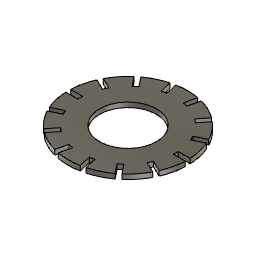
Assembly_file (Autodesk Fusion 360 archive; units mm, degrees)
design "Hringur_Litill"
Autodesk Fusion 360 part; units mm, degrees
sketch "Sketch1" plane through (0, 0, 0) normal (0, 0, 1) x (1, 0, 0)
  circle A0 centre (0, 0) radius 23.75
  line L0 (49.96, 2) -> (39.96, 2)
  line L1 (39.96, 2) -> (39.96, -2)
  line L2 (39.96, -2) -> (49.96, -2)
  line L3 (44.1446, 23.4788) -> (35.1349, 19.1399)
  line L4 (36.8705, 15.536) -> (45.8802, 19.8749)
  line L5 (35.1349, 19.1399) -> (36.8705, 15.536)
  line L6 (29.5859, 40.3073) -> (23.351, 32.489)
  line L7 (26.4783, 29.995) -> (32.7132, 37.8133)
  line L8 (23.351, 32.489) -> (26.4783, 29.995)
  line L9 (9.1673, 49.1524) -> (6.9421, 39.4031)
  line L10 (10.8418, 38.5131) -> (13.067, 48.2623)
  line L11 (6.9421, 39.4031) -> (10.8418, 38.5131)
  line L12 (-13.067, 48.2623) -> (-10.8418, 38.5131)
  line L13 (-6.9421, 39.4031) -> (-9.1673, 49.1524)
  line L14 (-10.8418, 38.5131) -> (-6.9421, 39.4031)
  line L15 (-32.7132, 37.8133) -> (-26.4783, 29.995)
  line L16 (-23.351, 32.489) -> (-29.5859, 40.3073)
  line L17 (-26.4783, 29.995) -> (-23.351, 32.489)
  line L18 (-45.8802, 19.8749) -> (-36.8705, 15.536)
  line L19 (-35.1349, 19.1399) -> (-44.1446, 23.4788)
  line L20 (-36.8705, 15.536) -> (-35.1349, 19.1399)
  line L21 (-49.96, -2) -> (-39.96, -2)
  line L22 (-39.96, 2) -> (-49.96, 2)
  line L23 (-39.96, -2) -> (-39.96, 2)
  line L24 (-44.1446, -23.4788) -> (-35.1349, -19.1399)
  line L25 (-36.8705, -15.536) -> (-45.8802, -19.8749)
  line L26 (-35.1349, -19.1399) -> (-36.8705, -15.536)
  line L27 (-29.5859, -40.3073) -> (-23.351, -32.489)
  line L28 (-26.4783, -29.995) -> (-32.7132, -37.8133)
  line L29 (-23.351, -32.489) -> (-26.4783, -29.995)
  line L30 (-9.1673, -49.1524) -> (-6.9421, -39.4031)
  line L31 (-10.8418, -38.5131) -> (-13.067, -48.2623)
  line L32 (-6.9421, -39.4031) -> (-10.8418, -38.5131)
  line L33 (13.067, -48.2623) -> (10.8418, -38.5131)
  line L34 (6.9421, -39.4031) -> (9.1673, -49.1524)
  line L35 (10.8418, -38.5131) -> (6.9421, -39.4031)
  line L36 (32.7132, -37.8133) -> (26.4783, -29.995)
  line L37 (23.351, -32.489) -> (29.5859, -40.3073)
  line L38 (26.4783, -29.995) -> (23.351, -32.489)
  line L39 (45.8802, -19.8749) -> (36.8705, -15.536)
  line L40 (35.1349, -19.1399) -> (44.1446, -23.4788)
  line L41 (36.8705, -15.536) -> (35.1349, -19.1399)
  arc A1 (49.96, 2) -> (45.8802, 19.8749) centre (0, 0) ccw
  arc A2 (44.1446, 23.4788) -> (32.7132, 37.8133) centre (0, 0) ccw
  arc A3 (29.5859, 40.3073) -> (13.067, 48.2623) centre (0, 0) ccw
  arc A4 (9.1673, 49.1524) -> (-9.1673, 49.1524) centre (0, 0) ccw
  arc A5 (-13.067, 48.2623) -> (-29.5859, 40.3073) centre (0, 0) ccw
  arc A6 (-32.7132, 37.8133) -> (-44.1446, 23.4788) centre (0, 0) ccw
  arc A7 (-45.8802, 19.8749) -> (-49.96, 2) centre (0, 0) ccw
  arc A8 (-49.96, -2) -> (-45.8802, -19.8749) centre (0, 0) ccw
  arc A9 (-44.1446, -23.4788) -> (-32.7132, -37.8133) centre (0, 0) ccw
  arc A10 (-29.5859, -40.3073) -> (-13.067, -48.2623) centre (0, 0) ccw
  arc A11 (-9.1673, -49.1524) -> (9.1673, -49.1524) centre (0, 0) ccw
  arc A12 (13.067, -48.2623) -> (29.5859, -40.3073) centre (0, 0) ccw
  arc A13 (32.7132, -37.8133) -> (44.1446, -23.4788) centre (0, 0) ccw
  arc A14 (45.8802, -19.8749) -> (49.96, -2) centre (0, 0) ccw
  dimension "d1" = 100
  dimension "d6" = 47.5
  dimension "d7" = 10
  dimension "d8" = 10
  dimension "d9" = 4
  dimension "d11" = 360
  constraint coincident A0.centre A1.centre
  constraint horizontal L0
  constraint perpendicular L0 L1
  constraint perpendicular L1 L2
  constraint concentric A1 A2
  constraint concentric A2 A3
  constraint concentric A3 A4
  constraint concentric A4 A5
  constraint concentric A5 A6
  constraint concentric A6 A7
  constraint concentric A7 A8
  constraint concentric A8 A9
  constraint concentric A9 A10
  constraint concentric A10 A11
  constraint concentric A11 A12
  constraint concentric A12 A13
  constraint concentric A13 A14
  measures "d1" diameter of A1
  measures "d6" diameter of A0
  measures "d7" distance of L0.start L0.end
  measures "d8" distance of L1.end L2.end
  measures "d9" distance of L0.end L1.end
extrude "Extrude1" add sketch "Sketch1" along normal blind 4
equation "d1 = D_o"
equation "D_o = 100 mm"
equation "D_i = 47.5 mm"
equation "þykkt = 4 mm"
equation "offset = 10 mm"
equation "d6 = D_i"
equation "d7 = offset"
equation "d8 = offset"
equation "d9 = þykkt"
equation "d12 = þykkt"

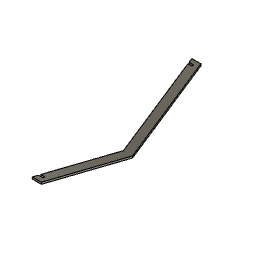
design "Lampi1"
Autodesk Fusion 360 part; units mm, degrees
sketch "Sketch1" plane through (0, 0, 0) normal (0, 0, 1) x (1, 0, 0)
  line L0 (0, 0) -> (20, 0)
  line L1 (20, 0) -> (120, -250)
  line L2 (120, -250) -> (70, -400)
  line L3 (70, -400) -> (50, -400)
  line L4 (4, -10) -> (14, -10)
  line L5 (53.3333, -390) -> (63.3333, -390)
  line L6 (63.3333, -386) -> (54.6667, -386)
  line L7 (100, -250) -> (54.6667, -386)
  line L8 (53.3333, -390) -> (50, -400)
  line L9 (0, 0) -> (4, -10)
  line L10 (5.6, -14) -> (100, -250)
  line L11 (14, -10) -> (14, -14)
  line L12 (5.6, -14) -> (14, -14)
  line L13 (63.3333, -390) -> (63.3333, -386)
  dimension "d4" = 400
  dimension "d5" = 50
  dimension "d6" = 50
  dimension "d7" = 250
  dimension "d9" = 20
  dimension "d10" = 20
  dimension "d11" = 20
  dimension "d12" = 10
  dimension "d13" = 4
  dimension "d14" = 10
  dimension "d15" = 10
  dimension "d16" = 4
  dimension "d17" = 10
  dimension "d27" = 4
  constraint coincident L0.start L9.start
  constraint horizontal L0
  constraint parallel L0 L3
  constraint parallel L1 L9
  constraint parallel L0 L4
  constraint coincident L10.start L9
  constraint coincident L5.start L7
  constraint parallel L3 L5
  constraint parallel L5 L6
  constraint collinear L7 L8
  constraint collinear L9 L10
  constraint perpendicular L11 L12
  constraint perpendicular L6 L13
  measures "d4" vertical distance of L0.start L3.end
  measures "d5" horizontal distance of L7.start L3.end
  measures "d6" horizontal distance of L0.start L3.end
  measures "d7" vertical distance of L0.start L7.start
  measures "d9" distance of L0.start L0.end
  measures "d10" distance of L7.start L1.end
  measures "d11" horizontal distance of L3.end L2.end
  measures "d12" vertical distance of L0.start L4.start
  measures "d13" vertical distance of L4.start L10.start
  measures "d14" distance of L4.start L4.end
  measures "d15" vertical distance of L3.end L5.start
  measures "d16" vertical distance of L5.start L6.end
  measures "d17" distance of L5.start L5.end
  measures "d27" distance of L4.end L11.end
extrude "Extrude1" add sketch "Sketch1" along normal blind 4
sketch "Sketch1 (2)" plane through (0, 0, 0) normal (0, 0, 1) x (1, 0, 0) in component "Lampi1"
component "Lampi1" placed x (1, 0, 0) y (0, 1, 0) z (0, 0, 1) at (0, 0, 0)
equation "d4 = haed_skerms"
equation "d5 = umfram_radius"
equation "d6 = umfram_radius"
equation "d7 = haed_u"
equation "d9 = þykkt_eining"
equation "d10 = þykkt_eining"
equation "d11 = þykkt_eining"
equation "d12 = dypt_pressfit"
equation "d13 = þykkt"
equation "d14 = dypt_pressfit"
equation "d15 = dypt_pressfit"
equation "d16 = þykkt"
equation "d17 = dypt_pressfit"
equation "haed_skerms = 400 mm"
equation "haed_u = 250 mm"
equation "head_l = 150 mm"
equation "þykkt = 4 mm"
equation "dypt_pressfit = 10 mm"
equation "umfram_radius = 50 mm"
equation "þykkt_eining = 20 mm"

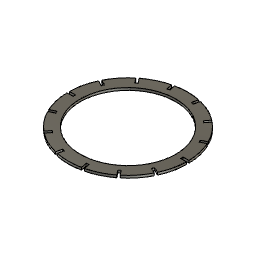
design "Hringur_Stor"
Autodesk Fusion 360 part; units mm, degrees
sketch "Sketch1" plane through (0, 0, 0) normal (0, 0, 1) x (1, 0, 0)
  circle A0 centre (0, 0) radius 80
  line L0 (99.98, 2) -> (89.98, 2)
  line L1 (89.98, 2) -> (89.98, -2)
  line L2 (89.98, -2) -> (99.98, -2)
  line L3 (89.2111, 45.1816) -> (80.2014, 40.8428)
  line L4 (81.9369, 37.2389) -> (90.9466, 41.5778)
  line L5 (80.2014, 40.8428) -> (81.9369, 37.2389)
  line L6 (60.7728, 79.4145) -> (54.5379, 71.5962)
  line L7 (57.6653, 69.1022) -> (63.9002, 76.9205)
  line L8 (54.5379, 71.5962) -> (57.6653, 69.1022)
  line L9 (20.2978, 97.9183) -> (18.0726, 88.1691)
  line L10 (21.9723, 87.279) -> (24.1975, 97.0282)
  line L11 (18.0726, 88.1691) -> (21.9723, 87.279)
  line L12 (-24.1975, 97.0282) -> (-21.9723, 87.279)
  line L13 (-18.0726, 88.1691) -> (-20.2978, 97.9183)
  line L14 (-21.9723, 87.279) -> (-18.0726, 88.1691)
  line L15 (-63.9002, 76.9205) -> (-57.6653, 69.1022)
  line L16 (-54.5379, 71.5962) -> (-60.7728, 79.4145)
  line L17 (-57.6653, 69.1022) -> (-54.5379, 71.5962)
  line L18 (-90.9466, 41.5778) -> (-81.9369, 37.2389)
  line L19 (-80.2014, 40.8428) -> (-89.2111, 45.1816)
  line L20 (-81.9369, 37.2389) -> (-80.2014, 40.8428)
  line L21 (-99.98, -2) -> (-89.98, -2)
  line L22 (-89.98, 2) -> (-99.98, 2)
  line L23 (-89.98, -2) -> (-89.98, 2)
  line L24 (-89.2111, -45.1816) -> (-80.2014, -40.8428)
  line L25 (-81.9369, -37.2389) -> (-90.9466, -41.5778)
  line L26 (-80.2014, -40.8428) -> (-81.9369, -37.2389)
  line L27 (-60.7728, -79.4145) -> (-54.5379, -71.5962)
  line L28 (-57.6653, -69.1022) -> (-63.9002, -76.9205)
  line L29 (-54.5379, -71.5962) -> (-57.6653, -69.1022)
  line L30 (-20.2978, -97.9183) -> (-18.0726, -88.1691)
  line L31 (-21.9723, -87.279) -> (-24.1975, -97.0282)
  line L32 (-18.0726, -88.1691) -> (-21.9723, -87.279)
  line L33 (24.1975, -97.0282) -> (21.9723, -87.279)
  line L34 (18.0726, -88.1691) -> (20.2978, -97.9183)
  line L35 (21.9723, -87.279) -> (18.0726, -88.1691)
  line L36 (63.9002, -76.9205) -> (57.6653, -69.1022)
  line L37 (54.5379, -71.5962) -> (60.7728, -79.4145)
  line L38 (57.6653, -69.1022) -> (54.5379, -71.5962)
  line L39 (90.9466, -41.5778) -> (81.9369, -37.2389)
  line L40 (80.2014, -40.8428) -> (89.2111, -45.1816)
  line L41 (81.9369, -37.2389) -> (80.2014, -40.8428)
  arc A1 (99.98, 2) -> (90.9466, 41.5778) centre (0, 0) ccw
  arc A2 (89.2111, 45.1816) -> (63.9002, 76.9205) centre (0, 0) ccw
  arc A3 (60.7728, 79.4145) -> (24.1975, 97.0282) centre (0, 0) ccw
  arc A4 (20.2978, 97.9183) -> (-20.2978, 97.9183) centre (0, 0) ccw
  arc A5 (-24.1975, 97.0282) -> (-60.7728, 79.4145) centre (0, 0) ccw
  arc A6 (-63.9002, 76.9205) -> (-89.2111, 45.1816) centre (0, 0) ccw
  arc A7 (-90.9466, 41.5778) -> (-99.98, 2) centre (0, 0) ccw
  arc A8 (-99.98, -2) -> (-90.9466, -41.5778) centre (0, 0) ccw
  arc A9 (-89.2111, -45.1816) -> (-63.9002, -76.9205) centre (0, 0) ccw
  arc A10 (90.9466, -41.5778) -> (99.98, -2) centre (0, 0) ccw
  arc A11 (63.9002, -76.9205) -> (89.2111, -45.1816) centre (0, 0) ccw
  arc A12 (24.1975, -97.0282) -> (60.7728, -79.4145) centre (0, 0) ccw
  arc A13 (-60.7728, -79.4145) -> (-24.1975, -97.0282) centre (0, 0) ccw
  arc A14 (-20.2978, -97.9183) -> (20.2978, -97.9183) centre (0, 0) ccw
  dimension "d1" = 200
  dimension "d2" = 160
  dimension "d5" = 4
  dimension "d6" = 10
  dimension "d7" = 10
  dimension "d13" = 360
  constraint coincident A0.centre A1.centre
  constraint horizontal L0
  constraint perpendicular L0 L1
  constraint perpendicular L1 L2
  constraint concentric A1 A2
  constraint concentric A2 A3
  constraint concentric A3 A4
  constraint concentric A4 A5
  constraint concentric A5 A6
  constraint concentric A6 A7
  constraint concentric A7 A8
  constraint concentric A8 A9
  constraint concentric A9 A13
  constraint concentric A10 A13
  constraint concentric A11 A13
  constraint concentric A12 A13
  constraint concentric A13 A14
  measures "d1" diameter of A1
  measures "d2" diameter of A0
  measures "d5" distance of L0.end L1.end
  measures "d6" distance of L0.start L0.end
  measures "d7" distance of L1.end L2.end
extrude "Extrude1" add sketch "Sketch1" along normal blind 4
component "Hringur_Stor" placed x (1, 0, 0) y (0, 1, 0) z (0, 0, 1) at (0, 0, 0)
equation "d1 = D_o"
equation "d2 = D_i"
equation "d5 = þykkt"
equation "d6 = dypt_pressfit"
equation "d7 = dypt_pressfit"
equation "D_o = 200 mm"
equation "D_i = 160 mm"
equation "dypt_pressfit = 10 mm"
equation "þykkt = 4 mm"
